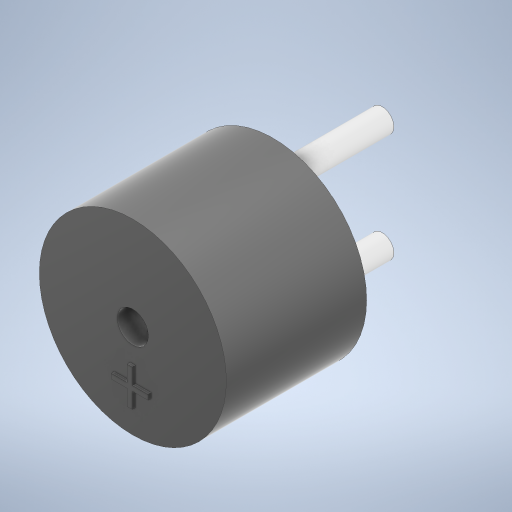
# Autodesk Inventor part: Buzzer
Saved by Autodesk Inventor 2024.3 (Build 283343000, 343)
## iProperties
Created: 2025-01-23
Part Number: Buzzer
Material: PBT Plastic
Document SubType Name: Modeling
Designer: ASUS TUF
Density: 1.31 g/cm^3
Appearance: Smooth - White
Author: ASUS TUF
Autodesk Inventor part; units mm, degrees
ref_plane "YZ Plane" through (0, 0, 0) normal (1, 0, 0) x (0, 1, 0)
ref_plane "XZ Plane" through (0, 0, 0) normal (0, 1, 0) x (-1, 0, 0)
ref_plane "XY Plane" through (0, 0, 0) normal (0, 0, 1) x (1, 0, 0)
sketch "Sketch1" plane through (0, 0, 0) normal (0, 0, 1) x (1, 0, 0)
  circle A0 centre (0, 0) radius 6
  dimension "d0" = 12
  constraints: 1 centre point, 1 coincident
  measures "d0" diameter of A0
extrude "Extrusion1" add sketch "Sketch1" along normal blind 9
sketch "Sketch2" plane through (0, 0, 9) normal (0, 0, 1) x (1, 0, 0)
  circle A0 centre (0, 0) radius 1
  line L0 (-2.0016, -1.6454) -> (2.0016, -1.6454) construction
  line L1 (2.0016, -1.6454) -> (2.0016, -4.7864) construction
  line L2 (2.0016, -4.7864) -> (-2.0016, -4.7864) construction
  line L3 (-2.0016, -4.7864) -> (-2.0016, -1.6454) construction
  line L4 (1.1852, -3.3776) -> (0.169, -3.3776)
  line L5 (0.169, -3.3776) -> (0.169, -4.3938)
  line L6 (0.169, -4.3938) -> (-0.1665, -4.3938)
  line L7 (-0.1665, -4.3938) -> (-0.1665, -3.3776)
  line L8 (-0.1665, -3.3776) -> (-1.1827, -3.3776)
  line L9 (-1.1827, -3.3776) -> (-1.1827, -3.0543)
  line L10 (-1.1827, -3.0543) -> (-0.1665, -3.0543)
  line L11 (-0.1665, -3.0543) -> (-0.1665, -2.0381)
  line L12 (-0.1665, -2.0381) -> (0.169, -2.0381)
  line L13 (0.169, -2.0381) -> (0.169, -3.0543)
  line L14 (0.169, -3.0543) -> (1.1852, -3.0543)
  line L15 (1.1852, -3.0543) -> (1.1852, -3.3776)
  point P0 (0, -1.6454)
  dimension "d3" = 2
  constraints: 1 centre point, 1 coincident, 1 midpoint, 1 vertical alignment, 2 other
  measures "d3" diameter of A0
extrude "Extrusion2" cut sketch "Sketch2" against normal blind 5 contours A0
extrude "Extrusion3" add sketch "Sketch2" along normal blind 0.2 contours L4 L5 L6 L7 L8 L9 L10 L11 L12 L13 L14 L15
sketch "Sketch3" plane through (0, 0, 0) normal (0, 0, -1) x (-1, 0, 0)
  circle A0 centre (0, 3.5) radius 0.75
  circle A1 centre (0, -3.5) radius 0.75
  line L0 (0, 3.5) -> (0, -3.5) construction
  point P0 (0, 0)
  point P1 (0, 0)
  dimension "d8" = 1.5
  dimension "d9" = 7
  constraints: 2 centre point, 2 end point, 2 vertical alignment, 1 coincident, 1 equal radius, 1 midpoint, 1 vertical
  measures "d8" diameter of A0
  measures "d9" distance of L0.start L0.end
extrude "Extrusion4" add sketch "Sketch3" along normal blind 7
body "Solid1"
